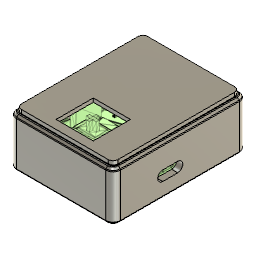
TapperS (Autodesk Fusion 360 design; units mm, degrees)
Autodesk Fusion 360 part; units mm, degrees
other "Base Mesh Feature1"
sketch "Sketch1" plane through (0, 0, 0) normal (0, 0, 1) x (1, 0, 0)
  line L0 (102, -120) -> (102, -123)
  line L1 (102, -123) -> (99, -123)
  line L2 (99, -123) -> (141, -123)
  line L3 (141, -123) -> (141, -69)
  line L4 (141, -69) -> (99, -69)
  line L5 (99, -69) -> (99, -123)
  line L6 (100.5, -121.5) -> (139.5, -121.5)
  line L7 (139.5, -121.5) -> (139.5, -70.5)
  line L8 (139.5, -70.5) -> (100.5, -70.5)
  line L9 (100.5, -70.5) -> (100.5, -121.5)
  line L10 (101.5, -120.5) -> (138.5, -120.5)
  line L11 (138.5, -120.5) -> (138.5, -71.5)
  line L12 (138.5, -71.5) -> (101.5, -71.5)
  line L13 (101.5, -71.5) -> (101.5, -120.5)
  line L14 (103, -120.5) -> (103, -71.5)
  line L15 (137, -71.5) -> (137, -120.5)
  dimension "d1" = 3
  dimension "d2" = 42
  dimension "d3" = 54
  dimension "d4" = 3
  dimension "d5" = -1.5
  dimension "d6" = -2.5
  dimension "d15" = 1.5
  dimension "d16" = 1.5
  constraint vertical L0
  constraint perpendicular L0 L1
  constraint horizontal L2
  constraint vertical L3
  constraint horizontal L4
  constraint vertical L5
  constraint coincident L10 L14.start
  constraint coincident L12 L14.end
  constraint perpendicular L12 L14
  constraint coincident L12 L15.start
  constraint coincident L10 L15.end
  constraint perpendicular L10 L15
  measures "d1" distance of L0.end L1.end
  measures "d2" distance of L1.end L2.end
  measures "d3" distance of L1.end L4.end
  measures "d4" distance of L0.start L0.end
  measures "d15" distance of L11 L15
  measures "d16" distance of L13 L14
extrude "Extrude1" add sketch "Sketch1" along normal blind 15 and the other way blind 5 contours L1 L2 L3 L4 L5 makes body 1
extrude "Extrude2" add sketch "Sketch1" along normal blind 13 and the other way blind 3 contours L6 L7 L8 L9 bodies 1
extrude "Extrude3" add sketch "Sketch1" against normal blind 2 contours L10 L12 L13 L14 | L10 L11 L12 L15 bodies 1
fillet "Fillet1" radius 3 4 edges at (141, -69, 5) (99, -69, 5) (141, -123, 5) (99, -123, 5) on bodies 1
fillet "Fillet2" radius 2 4 edges at (100.5, -121.5, -4) (139.5, -121.5, -4) (139.5, -70.5, -4) (100.5, -70.5, -4) on bodies 1
chamfer "Chamfer1" distance 1.5 angle 45 2 edges at (103, -96, -2) (137, -96, -2) on bodies 1
fillet "Fillet3" radius 2 4 edges at (100.5, -70.5, 14) (139.5, -70.5, 14) (139.5, -121.5, 14) (100.5, -121.5, 14) on bodies 1
chamfer "Chamfer2" distance 1 angle 45 16 edges at (99, -96, 15) (99.8787, -122.1213, 15) (120, -123, 15) (140.1213, -122.1213, 15) (141, -96, 15) (140.1213, -69.8787, 15) (120, -69, 15) (99.8787, -69.8787, 15) (99, -96, -5) (99.8787, -69.8787, -5) (120, -69, -5) (140.1213, -69.8787, -5) (141, -96, -5) (140.1213, -122.1213, -5) (120, -123, -5) (99.8787, -122.1213, -5) on bodies 1
fillet "Fillet4" radius 0.5 16 edges at (120, -123, 14) (140.1213, -122.1213, 14) (141, -96, 14) (140.1213, -69.8787, 14) (120, -69, 14) (99.8787, -69.8787, 14) (99, -96, 14) (99.8787, -122.1213, 14) (120, -70, 15) (139.4142, -70.5858, 15) (140, -96, 15) (139.4142, -121.4142, 15) (120, -122, 15) (100.5858, -121.4142, 15) (100, -96, 15) (100.5858, -70.5858, 15) on bodies 1
fillet "Fillet4" radius 0.5 16 edges at (120, -69, -4) (140.1213, -69.8787, -4) (141, -96, -4) (140.1213, -122.1213, -4) (120, -123, -4) (99.8787, -122.1213, -4) (99, -96, -4) (99.8787, -69.8787, -4) (120, -122, -5) (139.4142, -121.4142, -5) (140, -96, -5) (139.4142, -70.5858, -5) (120, -70, -5) (100.5858, -70.5858, -5) (100, -96, -5) (100.5858, -121.4142, -5) on bodies 1
sketch "Sketch2" plane through (138.5, 0, 0) normal (-1, 0, 0) x (0, -1, 0)
  line L0 (71.5, 0) -> (120.5, 0)
  line L1 (120.5, 0) -> (120.5, 13)
  line L2 (120.5, 13) -> (71.5, 13)
  line L3 (71.5, 13) -> (71.5, 0)
  line L4 (102.9827, 5.3365) -> (96.9293, 5.3365)
  arc A0 (96.9293, 5.3365) -> (96.9293, 1.3132) centre (96.9293, 3.3249) ccw
  line L5 (96.9293, 1.3132) -> (102.9827, 1.3132)
  arc A1 (102.9827, 1.3132) -> (102.9827, 5.3365) centre (102.9827, 3.3249) ccw
  line L6 (102.9827, 3.3249) -> (96.9293, 3.3249) construction
  arc A2 (96.9293, 7.3365) -> (96.9293, -0.6868) centre (96.9293, 3.3249) ccw
  line L7 (96.9293, -0.6868) -> (102.9827, -0.6868)
  arc A3 (102.9827, -0.6868) -> (102.9827, 7.3365) centre (102.9827, 3.3249) ccw
  line L8 (102.9827, 7.3365) -> (96.9293, 7.3365)
  dimension "d33" = 2
  constraint tangent L4 A0
  constraint tangent A0 L5
  constraint parallel L4 L5
  constraint tangent L5 A1
  constraint tangent L4 A1
  constraint horizontal L6
extrude "Extrude4" cut sketch "Sketch2" against normal blind 3.5 contours L4 A0 L5 A1 bodies 1
sketch "Sketch3" plane through (0, 0, 15) normal (0, 0, 1) x (-1, 0, 0)
  line L0 (-100.5, 119.5) -> (-100.5, 72.5)
  arc A0 (-102.5, 70.5) -> (-100.5, 72.5) centre (-102.5, 72.5) ccw
  line L1 (-102.5, 70.5) -> (-137.5, 70.5)
  arc A1 (-139.5, 72.5) -> (-137.5, 70.5) centre (-137.5, 72.5) ccw
  line L2 (-139.5, 72.5) -> (-139.5, 119.5)
  arc A2 (-137.5, 121.5) -> (-139.5, 119.5) centre (-137.5, 119.5) ccw
  line L3 (-137.5, 121.5) -> (-102.5, 121.5)
  arc A3 (-100.5, 119.5) -> (-102.5, 121.5) centre (-102.5, 119.5) ccw
  line L4 (-138, 70.2071) -> (-102, 70.2071)
  arc A4 (-102, 70.2071) -> (-100.2071, 72) centre (-102, 72) ccw
  line L5 (-100.2071, 72) -> (-100.2071, 120)
  arc A5 (-100.2071, 120) -> (-102, 121.7929) centre (-102, 120) ccw
  line L6 (-102, 121.7929) -> (-138, 121.7929)
  arc A6 (-138, 121.7929) -> (-139.7929, 120) centre (-138, 120) ccw
  line L7 (-139.7929, 120) -> (-139.7929, 72)
  arc A7 (-139.7929, 72) -> (-138, 70.2071) centre (-138, 72) ccw
  line L8 (-113, 103) -> (-128, 103)
  line L9 (-128, 103) -> (-128, 118)
  line L10 (-128, 118) -> (-113, 118)
  line L11 (-113, 118) -> (-113, 103)
  constraint horizontal L8
  constraint vertical L9
  constraint horizontal L10
  constraint vertical L11
extrude "Extrude5" add sketch "Sketch3" along normal blind 1.5 separate body contours L0 A0 L1 A1 L2 A2 L3 A3 | L8 L9 L10 L11 makes body 2
extrude "Extrude6" cut sketch "Sketch3" along normal blind 2 contours L8 L9 L10 L11 bodies 2
